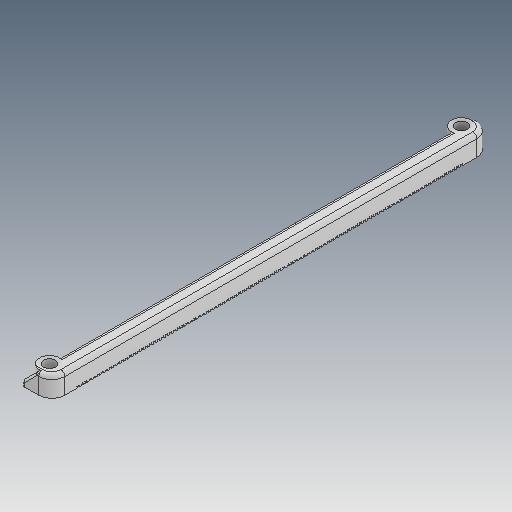
# Autodesk Inventor part: front_panel_mount_end
Saved by Autodesk Inventor 2027 (Build 310192060, 192F)
## iProperties
Created: 2026-07-28
Part Number: front_panel_mount_end
Material: Generic
Document SubType Name: Modeling
Designer: prest
Density: 1 g/cm^3
Appearance: Default
Author: prest
Autodesk Inventor part; units mm, degrees
ref_plane "YZ Plane" through (0, 0, 0) normal (1, 0, 0) x (0, 1, 0)
ref_plane "XZ Plane" through (0, 0, 0) normal (0, 1, 0) x (-1, 0, 0)
ref_plane "XY Plane" through (0, 0, 0) normal (0, 0, 1) x (1, 0, 0)
sketch "Sketch1" plane through (0, 0, 0) normal (0, 1, 0) x (-1, 0, 0)
  line L0 (7.375, 108.5) -> (-7.375, 108.5)
  line L1 (-7.375, 108.5) -> (-7.375, -108.5)
  line L2 (-7.375, -108.5) -> (7.375, -108.5)
  line L3 (7.375, -108.5) -> (7.375, 108.5)
  point P0 (0, 0)
  point P1 (0, 108.5)
  point P2 (7.375, 0)
  dimension "d0" = 217
  dimension "d1" = 14.75
  constraints: 8 end point, 2 midpoint, 2 parallel, 1 horizontal, 1 horizontal alignment, 1 perpendicular, 1 vertical alignment
  measures "d0" distance of L2.end L0.start
  measures "d1" distance of L0.start L0.end
extrude "Extrusion1" add sketch "Sketch1" along normal blind 10
chamfer "Chamfer1" distance 8 angle 45 1 edges at (-7.375, 10, 0)
sketch "Sketch2" plane through (0, 0, 0) normal (0, -1, 0) x (1, 0, 0)
  line L0 (-7.375, -108.5) -> (-7.375, 108.5) projected
  point P0 (0, 0)
  point P1 (0.068, -101.6793)
  point P2 (0.068, 102.3207)
  point P3 (-7.375, -108.4123)
  point P4 (-7.375, 108.4123)
  dimension "d10" = 204
  dimension "d11" = 7.443
  constraints: 1 vertical alignment
  measures "d10" distance of point (0.068, -101.679) point (0.068, 102.321)
  measures "d11" distance from line of L0 point (0.068, 102.321)
hole "Hole1" at (0.068, 0, -101.6793) at (0.068, 0, 102.3207) direction (0, 1, 0) diameter 6 end through all
sketch "Sketch3" plane through (0, 0, 0) normal (0, -1, 0) x (1, 0, 0)
  arc A0 (0.625, -98.7315) -> (0.625, -104.6271) centre (0.068, -101.6793) ccw projected
  circle A1 centre (0.068, -101.6793) radius 3
  circle A2 centre (0.068, -101.6793) radius 5
  circle A3 centre (0.068, 102.3207) radius 3 projected
  circle A4 centre (0.068, 102.3207) radius 5
  point P0 (0, 0)
  point P1 (0.0392, -98.6794)
  point P2 (0.0392, -104.6792)
  point P3 (0.0392, -104.6792)
  point P4 (0.0392, -98.6794)
  dimension "d19" = 10
  dimension "d20" = 10
  constraints: 3 centre point, 3 coincident
  measures "d19" diameter of A2
  measures "d20" diameter of A4
extrude "Extrusion2" add sketch "Sketch3" against normal blind 10
fillet "Fillet5" radius 6.5 2 edges at (7.375, 5, 108.5) (7.375, 5, -108.5)
fillet "Fillet6" radius 2 6 edges at (0.75, 10, 108.5) (7.375, 10, 0) (5.4712, 10, -106.5962) (0.75, 10, -108.5) (5.4712, 10, 106.5962) (0.625, 10, 0.3207)
fillet "Fillet7" radius 2 1 edges at (-7.375, 2, 0)
fillet "Fillet8" radius 1 8 edges at (-0.2821, 9.0929, 108.175) (-7.2228, 1.9369, 108.5) (-7.375, 0.5858, 108.5) (-4.0821, 5.2929, 108.5) (-7.2228, 1.9369, -108.5) (-7.375, 0.5858, -108.5) (-0.0144, 9.3606, -107.9659) (-4.0821, 5.2929, -108.5)
sketch "Sketch4" plane through (0.0392, 9.4142, -96.6794) normal (-0.7071068, 0.7071068, 0) x (-0.7071068, -0.7071068, 0)
  line L0 (8.6569, 192.6794) -> (1, 192.6794)
  line L1 (1, 191.6794) -> (8.6569, 191.6794)
  line L2 (8.6569, 191.6794) -> (8.6569, 192.6794)
  line L3 (1, 192.6794) -> (1, 191.6794)
  line L4 (1, -11.8206) -> (9.6569, -11.8206) projected
  ellipse E0 centre (6.6365, -4.9999) end of major axis (6.6365, -7.9999) minor radius 2.1213 projected
  line L5 (-6.7225, 1.1794) -> (12.4454, 1.1794) construction
  line L6 (11.8995, -10.8206) -> (11.8995, 204.1794) projected
  line L7 (9.6569, 205.1794) -> (1, 205.1794) projected
  line L8 (0, 0) -> (0, 194.0002) projected
  line L9 (9.6569, 204.1794) -> (9.6569, -10.8206) projected
  line L10 (8.6569, 190.6794) -> (1, 190.6794)
  line L11 (8.6569, 189.6794) -> (8.6569, 190.6794)
  line L12 (1, 189.6794) -> (8.6569, 189.6794)
  line L13 (1, 190.6794) -> (1, 189.6794)
  line L14 (8.6569, 188.6794) -> (1, 188.6794)
  line L15 (8.6569, 187.6794) -> (8.6569, 188.6794)
  line L16 (1, 187.6794) -> (8.6569, 187.6794)
  line L17 (1, 188.6794) -> (1, 187.6794)
  line L18 (8.6569, 186.6794) -> (1, 186.6794)
  line L19 (8.6569, 185.6794) -> (8.6569, 186.6794)
  line L20 (1, 185.6794) -> (8.6569, 185.6794)
  line L21 (1, 186.6794) -> (1, 185.6794)
  line L22 (8.6569, 184.6794) -> (1, 184.6794)
  line L23 (8.6569, 183.6794) -> (8.6569, 184.6794)
  line L24 (1, 183.6794) -> (8.6569, 183.6794)
  line L25 (1, 184.6794) -> (1, 183.6794)
  line L26 (8.6569, 182.6794) -> (1, 182.6794)
  line L27 (8.6569, 181.6794) -> (8.6569, 182.6794)
  line L28 (1, 181.6794) -> (8.6569, 181.6794)
  line L29 (1, 182.6794) -> (1, 181.6794)
  line L30 (8.6569, 180.6794) -> (1, 180.6794)
  line L31 (8.6569, 179.6794) -> (8.6569, 180.6794)
  line L32 (1, 179.6794) -> (8.6569, 179.6794)
  line L33 (1, 180.6794) -> (1, 179.6794)
  line L34 (8.6569, 178.6794) -> (1, 178.6794)
  line L35 (8.6569, 177.6794) -> (8.6569, 178.6794)
  line L36 (1, 177.6794) -> (8.6569, 177.6794)
  line L37 (1, 178.6794) -> (1, 177.6794)
  line L38 (8.6569, 176.6794) -> (1, 176.6794)
  line L39 (8.6569, 175.6794) -> (8.6569, 176.6794)
  line L40 (1, 175.6794) -> (8.6569, 175.6794)
  line L41 (1, 176.6794) -> (1, 175.6794)
  line L42 (8.6569, 174.6794) -> (1, 174.6794)
  line L43 (8.6569, 173.6794) -> (8.6569, 174.6794)
  line L44 (1, 173.6794) -> (8.6569, 173.6794)
  line L45 (1, 174.6794) -> (1, 173.6794)
  line L46 (8.6569, 172.6794) -> (1, 172.6794)
  line L47 (8.6569, 171.6794) -> (8.6569, 172.6794)
  line L48 (1, 171.6794) -> (8.6569, 171.6794)
  line L49 (1, 172.6794) -> (1, 171.6794)
  line L50 (8.6569, 170.6794) -> (1, 170.6794)
  line L51 (8.6569, 169.6794) -> (8.6569, 170.6794)
  line L52 (1, 169.6794) -> (8.6569, 169.6794)
  line L53 (1, 170.6794) -> (1, 169.6794)
  line L54 (8.6569, 168.6794) -> (1, 168.6794)
  line L55 (8.6569, 167.6794) -> (8.6569, 168.6794)
  line L56 (1, 167.6794) -> (8.6569, 167.6794)
  line L57 (1, 168.6794) -> (1, 167.6794)
  line L58 (8.6569, 166.6794) -> (1, 166.6794)
  line L59 (8.6569, 165.6794) -> (8.6569, 166.6794)
  line L60 (1, 165.6794) -> (8.6569, 165.6794)
  line L61 (1, 166.6794) -> (1, 165.6794)
  line L62 (8.6569, 164.6794) -> (1, 164.6794)
  line L63 (8.6569, 163.6794) -> (8.6569, 164.6794)
  line L64 (1, 163.6794) -> (8.6569, 163.6794)
  line L65 (1, 164.6794) -> (1, 163.6794)
  line L66 (8.6569, 162.6794) -> (1, 162.6794)
  line L67 (8.6569, 161.6794) -> (8.6569, 162.6794)
  line L68 (1, 161.6794) -> (8.6569, 161.6794)
  line L69 (1, 162.6794) -> (1, 161.6794)
  line L70 (8.6569, 160.6794) -> (1, 160.6794)
  line L71 (8.6569, 159.6794) -> (8.6569, 160.6794)
  line L72 (1, 159.6794) -> (8.6569, 159.6794)
  line L73 (1, 160.6794) -> (1, 159.6794)
  line L74 (8.6569, 158.6794) -> (1, 158.6794)
  line L75 (8.6569, 157.6794) -> (8.6569, 158.6794)
  line L76 (1, 157.6794) -> (8.6569, 157.6794)
  line L77 (1, 158.6794) -> (1, 157.6794)
  line L78 (8.6569, 156.6794) -> (1, 156.6794)
  line L79 (8.6569, 155.6794) -> (8.6569, 156.6794)
  line L80 (1, 155.6794) -> (8.6569, 155.6794)
  line L81 (1, 156.6794) -> (1, 155.6794)
  line L82 (8.6569, 154.6794) -> (1, 154.6794)
  line L83 (8.6569, 153.6794) -> (8.6569, 154.6794)
  line L84 (1, 153.6794) -> (8.6569, 153.6794)
  line L85 (1, 154.6794) -> (1, 153.6794)
  line L86 (8.6569, 152.6794) -> (1, 152.6794)
  line L87 (8.6569, 151.6794) -> (8.6569, 152.6794)
  line L88 (1, 151.6794) -> (8.6569, 151.6794)
  line L89 (1, 152.6794) -> (1, 151.6794)
  line L90 (8.6569, 150.6794) -> (1, 150.6794)
  line L91 (8.6569, 149.6794) -> (8.6569, 150.6794)
  line L92 (1, 149.6794) -> (8.6569, 149.6794)
  line L93 (1, 150.6794) -> (1, 149.6794)
  line L94 (8.6569, 148.6794) -> (1, 148.6794)
  line L95 (8.6569, 147.6794) -> (8.6569, 148.6794)
  line L96 (1, 147.6794) -> (8.6569, 147.6794)
  line L97 (1, 148.6794) -> (1, 147.6794)
  line L98 (8.6569, 146.6794) -> (1, 146.6794)
  line L99 (8.6569, 145.6794) -> (8.6569, 146.6794)
  line L100 (1, 145.6794) -> (8.6569, 145.6794)
  line L101 (1, 146.6794) -> (1, 145.6794)
  line L102 (8.6569, 144.6794) -> (1, 144.6794)
  line L103 (8.6569, 143.6794) -> (8.6569, 144.6794)
  line L104 (1, 143.6794) -> (8.6569, 143.6794)
  line L105 (1, 144.6794) -> (1, 143.6794)
  line L106 (8.6569, 142.6794) -> (1, 142.6794)
  line L107 (8.6569, 141.6794) -> (8.6569, 142.6794)
  line L108 (1, 141.6794) -> (8.6569, 141.6794)
  line L109 (1, 142.6794) -> (1, 141.6794)
  line L110 (8.6569, 140.6794) -> (1, 140.6794)
  line L111 (8.6569, 139.6794) -> (8.6569, 140.6794)
  line L112 (1, 139.6794) -> (8.6569, 139.6794)
  line L113 (1, 140.6794) -> (1, 139.6794)
  line L114 (8.6569, 138.6794) -> (1, 138.6794)
  line L115 (8.6569, 137.6794) -> (8.6569, 138.6794)
  line L116 (1, 137.6794) -> (8.6569, 137.6794)
  line L117 (1, 138.6794) -> (1, 137.6794)
  line L118 (8.6569, 136.6794) -> (1, 136.6794)
  line L119 (8.6569, 135.6794) -> (8.6569, 136.6794)
  line L120 (1, 135.6794) -> (8.6569, 135.6794)
  line L121 (1, 136.6794) -> (1, 135.6794)
  line L122 (8.6569, 134.6794) -> (1, 134.6794)
  line L123 (8.6569, 133.6794) -> (8.6569, 134.6794)
  line L124 (1, 133.6794) -> (8.6569, 133.6794)
  line L125 (1, 134.6794) -> (1, 133.6794)
  line L126 (8.6569, 132.6794) -> (1, 132.6794)
  line L127 (8.6569, 131.6794) -> (8.6569, 132.6794)
  line L128 (1, 131.6794) -> (8.6569, 131.6794)
  line L129 (1, 132.6794) -> (1, 131.6794)
  line L130 (8.6569, 130.6794) -> (1, 130.6794)
  line L131 (8.6569, 129.6794) -> (8.6569, 130.6794)
  line L132 (1, 129.6794) -> (8.6569, 129.6794)
  line L133 (1, 130.6794) -> (1, 129.6794)
  line L134 (8.6569, 128.6794) -> (1, 128.6794)
  line L135 (8.6569, 127.6794) -> (8.6569, 128.6794)
  line L136 (1, 127.6794) -> (8.6569, 127.6794)
  line L137 (1, 128.6794) -> (1, 127.6794)
  line L138 (8.6569, 126.6794) -> (1, 126.6794)
  line L139 (8.6569, 125.6794) -> (8.6569, 126.6794)
  line L140 (1, 125.6794) -> (8.6569, 125.6794)
  line L141 (1, 126.6794) -> (1, 125.6794)
  line L142 (8.6569, 124.6794) -> (1, 124.6794)
  line L143 (8.6569, 123.6794) -> (8.6569, 124.6794)
  line L144 (1, 123.6794) -> (8.6569, 123.6794)
  line L145 (1, 124.6794) -> (1, 123.6794)
  line L146 (8.6569, 122.6794) -> (1, 122.6794)
  line L147 (8.6569, 121.6794) -> (8.6569, 122.6794)
  line L148 (1, 121.6794) -> (8.6569, 121.6794)
  line L149 (1, 122.6794) -> (1, 121.6794)
  line L150 (8.6569, 120.6794) -> (1, 120.6794)
  line L151 (8.6569, 119.6794) -> (8.6569, 120.6794)
  line L152 (1, 119.6794) -> (8.6569, 119.6794)
  line L153 (1, 120.6794) -> (1, 119.6794)
  line L154 (8.6569, 118.6794) -> (1, 118.6794)
  line L155 (8.6569, 117.6794) -> (8.6569, 118.6794)
  line L156 (1, 117.6794) -> (8.6569, 117.6794)
  line L157 (1, 118.6794) -> (1, 117.6794)
  line L158 (8.6569, 116.6794) -> (1, 116.6794)
  line L159 (8.6569, 115.6794) -> (8.6569, 116.6794)
  line L160 (1, 115.6794) -> (8.6569, 115.6794)
  line L161 (1, 116.6794) -> (1, 115.6794)
  line L162 (8.6569, 114.6794) -> (1, 114.6794)
  line L163 (8.6569, 113.6794) -> (8.6569, 114.6794)
  line L164 (1, 113.6794) -> (8.6569, 113.6794)
  line L165 (1, 114.6794) -> (1, 113.6794)
  line L166 (8.6569, 112.6794) -> (1, 112.6794)
  line L167 (8.6569, 111.6794) -> (8.6569, 112.6794)
  line L168 (1, 111.6794) -> (8.6569, 111.6794)
  line L169 (1, 112.6794) -> (1, 111.6794)
  line L170 (8.6569, 110.6794) -> (1, 110.6794)
  line L171 (8.6569, 109.6794) -> (8.6569, 110.6794)
  line L172 (1, 109.6794) -> (8.6569, 109.6794)
  line L173 (1, 110.6794) -> (1, 109.6794)
  line L174 (8.6569, 108.6794) -> (1, 108.6794)
  line L175 (8.6569, 107.6794) -> (8.6569, 108.6794)
  line L176 (1, 107.6794) -> (8.6569, 107.6794)
  line L177 (1, 108.6794) -> (1, 107.6794)
  line L178 (8.6569, 106.6794) -> (1, 106.6794)
  line L179 (8.6569, 105.6794) -> (8.6569, 106.6794)
  line L180 (1, 105.6794) -> (8.6569, 105.6794)
  line L181 (1, 106.6794) -> (1, 105.6794)
  line L182 (8.6569, 104.6794) -> (1, 104.6794)
  line L183 (8.6569, 103.6794) -> (8.6569, 104.6794)
  line L184 (1, 103.6794) -> (8.6569, 103.6794)
  line L185 (1, 104.6794) -> (1, 103.6794)
  line L186 (8.6569, 102.6794) -> (1, 102.6794)
  line L187 (8.6569, 101.6794) -> (8.6569, 102.6794)
  line L188 (1, 101.6794) -> (8.6569, 101.6794)
  line L189 (1, 102.6794) -> (1, 101.6794)
  line L190 (8.6569, 100.6794) -> (1, 100.6794)
  line L191 (8.6569, 99.6794) -> (8.6569, 100.6794)
  line L192 (1, 99.6794) -> (8.6569, 99.6794)
  line L193 (1, 100.6794) -> (1, 99.6794)
  line L194 (8.6569, 98.6794) -> (1, 98.6794)
  line L195 (8.6569, 97.6794) -> (8.6569, 98.6794)
  line L196 (1, 97.6794) -> (8.6569, 97.6794)
  line L197 (1, 98.6794) -> (1, 97.6794)
  line L198 (8.6569, 96.6794) -> (1, 96.6794)
  line L199 (8.6569, 95.6794) -> (8.6569, 96.6794)
  line L200 (1, 95.6794) -> (8.6569, 95.6794)
  line L201 (1, 96.6794) -> (1, 95.6794)
  line L202 (8.6569, 94.6794) -> (1, 94.6794)
  line L203 (8.6569, 93.6794) -> (8.6569, 94.6794)
  line L204 (1, 93.6794) -> (8.6569, 93.6794)
  line L205 (1, 94.6794) -> (1, 93.6794)
  line L206 (8.6569, 92.6794) -> (1, 92.6794)
  line L207 (8.6569, 91.6794) -> (8.6569, 92.6794)
  line L208 (1, 91.6794) -> (8.6569, 91.6794)
  line L209 (1, 92.6794) -> (1, 91.6794)
  line L210 (8.6569, 90.6794) -> (1, 90.6794)
  line L211 (8.6569, 89.6794) -> (8.6569, 90.6794)
  line L212 (1, 89.6794) -> (8.6569, 89.6794)
  line L213 (1, 90.6794) -> (1, 89.6794)
  line L214 (8.6569, 88.6794) -> (1, 88.6794)
  line L215 (8.6569, 87.6794) -> (8.6569, 88.6794)
  line L216 (1, 87.6794) -> (8.6569, 87.6794)
  line L217 (1, 88.6794) -> (1, 87.6794)
  line L218 (8.6569, 86.6794) -> (1, 86.6794)
  line L219 (8.6569, 85.6794) -> (8.6569, 86.6794)
  line L220 (1, 85.6794) -> (8.6569, 85.6794)
  line L221 (1, 86.6794) -> (1, 85.6794)
  line L222 (8.6569, 84.6794) -> (1, 84.6794)
  line L223 (8.6569, 83.6794) -> (8.6569, 84.6794)
  line L224 (1, 83.6794) -> (8.6569, 83.6794)
  line L225 (1, 84.6794) -> (1, 83.6794)
  line L226 (8.6569, 82.6794) -> (1, 82.6794)
  line L227 (8.6569, 81.6794) -> (8.6569, 82.6794)
  line L228 (1, 81.6794) -> (8.6569, 81.6794)
  line L229 (1, 82.6794) -> (1, 81.6794)
  line L230 (8.6569, 80.6794) -> (1, 80.6794)
  line L231 (8.6569, 79.6794) -> (8.6569, 80.6794)
  line L232 (1, 79.6794) -> (8.6569, 79.6794)
  line L233 (1, 80.6794) -> (1, 79.6794)
  line L234 (8.6569, 78.6794) -> (1, 78.6794)
  line L235 (8.6569, 77.6794) -> (8.6569, 78.6794)
  line L236 (1, 77.6794) -> (8.6569, 77.6794)
  line L237 (1, 78.6794) -> (1, 77.6794)
  line L238 (8.6569, 76.6794) -> (1, 76.6794)
  line L239 (8.6569, 75.6794) -> (8.6569, 76.6794)
  line L240 (1, 75.6794) -> (8.6569, 75.6794)
  line L241 (1, 76.6794) -> (1, 75.6794)
  line L242 (8.6569, 74.6794) -> (1, 74.6794)
  line L243 (8.6569, 73.6794) -> (8.6569, 74.6794)
  line L244 (1, 73.6794) -> (8.6569, 73.6794)
  line L245 (1, 74.6794) -> (1, 73.6794)
  line L246 (8.6569, 72.6794) -> (1, 72.6794)
  line L247 (8.6569, 71.6794) -> (8.6569, 72.6794)
  line L248 (1, 71.6794) -> (8.6569, 71.6794)
  line L249 (1, 72.6794) -> (1, 71.6794)
  line L250 (8.6569, 70.6794) -> (1, 70.6794)
  line L251 (8.6569, 69.6794) -> (8.6569, 70.6794)
  line L252 (1, 69.6794) -> (8.6569, 69.6794)
  line L253 (1, 70.6794) -> (1, 69.6794)
  line L254 (8.6569, 68.6794) -> (1, 68.6794)
  line L255 (8.6569, 67.6794) -> (8.6569, 68.6794)
  line L256 (1, 67.6794) -> (8.6569, 67.6794)
  line L257 (1, 68.6794) -> (1, 67.6794)
  line L258 (8.6569, 66.6794) -> (1, 66.6794)
  line L259 (8.6569, 65.6794) -> (8.6569, 66.6794)
  line L260 (1, 65.6794) -> (8.6569, 65.6794)
  line L261 (1, 66.6794) -> (1, 65.6794)
  line L262 (8.6569, 64.6794) -> (1, 64.6794)
  line L263 (8.6569, 63.6794) -> (8.6569, 64.6794)
  line L264 (1, 63.6794) -> (8.6569, 63.6794)
  line L265 (1, 64.6794) -> (1, 63.6794)
  line L266 (8.6569, 62.6794) -> (1, 62.6794)
  line L267 (8.6569, 61.6794) -> (8.6569, 62.6794)
  line L268 (1, 61.6794) -> (8.6569, 61.6794)
  line L269 (1, 62.6794) -> (1, 61.6794)
  line L270 (8.6569, 60.6794) -> (1, 60.6794)
  line L271 (8.6569, 59.6794) -> (8.6569, 60.6794)
  line L272 (1, 59.6794) -> (8.6569, 59.6794)
  line L273 (1, 60.6794) -> (1, 59.6794)
  line L274 (8.6569, 58.6794) -> (1, 58.6794)
  line L275 (8.6569, 57.6794) -> (8.6569, 58.6794)
  line L276 (1, 57.6794) -> (8.6569, 57.6794)
  line L277 (1, 58.6794) -> (1, 57.6794)
  line L278 (8.6569, 56.6794) -> (1, 56.6794)
  line L279 (8.6569, 55.6794) -> (8.6569, 56.6794)
  line L280 (1, 55.6794) -> (8.6569, 55.6794)
  line L281 (1, 56.6794) -> (1, 55.6794)
  line L282 (8.6569, 54.6794) -> (1, 54.6794)
  line L283 (8.6569, 53.6794) -> (8.6569, 54.6794)
  line L284 (1, 53.6794) -> (8.6569, 53.6794)
  line L285 (1, 54.6794) -> (1, 53.6794)
  line L286 (8.6569, 52.6794) -> (1, 52.6794)
  line L287 (8.6569, 51.6794) -> (8.6569, 52.6794)
  line L288 (1, 51.6794) -> (8.6569, 51.6794)
  line L289 (1, 52.6794) -> (1, 51.6794)
  line L290 (8.6569, 50.6794) -> (1, 50.6794)
  line L291 (8.6569, 49.6794) -> (8.6569, 50.6794)
  line L292 (1, 49.6794) -> (8.6569, 49.6794)
  line L293 (1, 50.6794) -> (1, 49.6794)
  line L294 (8.6569, 48.6794) -> (1, 48.6794)
  line L295 (8.6569, 47.6794) -> (8.6569, 48.6794)
  line L296 (1, 47.6794) -> (8.6569, 47.6794)
  line L297 (1, 48.6794) -> (1, 47.6794)
  line L298 (8.6569, 46.6794) -> (1, 46.6794)
  line L299 (8.6569, 45.6794) -> (8.6569, 46.6794)
  line L300 (1, 45.6794) -> (8.6569, 45.6794)
  line L301 (1, 46.6794) -> (1, 45.6794)
  line L302 (8.6569, 44.6794) -> (1, 44.6794)
  line L303 (8.6569, 43.6794) -> (8.6569, 44.6794)
  line L304 (1, 43.6794) -> (8.6569, 43.6794)
  line L305 (1, 44.6794) -> (1, 43.6794)
  line L306 (8.6569, 42.6794) -> (1, 42.6794)
  line L307 (8.6569, 41.6794) -> (8.6569, 42.6794)
  line L308 (1, 41.6794) -> (8.6569, 41.6794)
  line L309 (1, 42.6794) -> (1, 41.6794)
  line L310 (8.6569, 40.6794) -> (1, 40.6794)
  line L311 (8.6569, 39.6794) -> (8.6569, 40.6794)
  line L312 (1, 39.6794) -> (8.6569, 39.6794)
  line L313 (1, 40.6794) -> (1, 39.6794)
  line L314 (8.6569, 38.6794) -> (1, 38.6794)
  line L315 (8.6569, 37.6794) -> (8.6569, 38.6794)
  line L316 (1, 37.6794) -> (8.6569, 37.6794)
  line L317 (1, 38.6794) -> (1, 37.6794)
  line L318 (8.6569, 36.6794) -> (1, 36.6794)
  line L319 (8.6569, 35.6794) -> (8.6569, 36.6794)
  line L320 (1, 35.6794) -> (8.6569, 35.6794)
  line L321 (1, 36.6794) -> (1, 35.6794)
  line L322 (8.6569, 34.6794) -> (1, 34.6794)
  line L323 (8.6569, 33.6794) -> (8.6569, 34.6794)
  line L324 (1, 33.6794) -> (8.6569, 33.6794)
  line L325 (1, 34.6794) -> (1, 33.6794)
  line L326 (8.6569, 32.6794) -> (1, 32.6794)
  line L327 (8.6569, 31.6794) -> (8.6569, 32.6794)
  line L328 (1, 31.6794) -> (8.6569, 31.6794)
  line L329 (1, 32.6794) -> (1, 31.6794)
  line L330 (8.6569, 30.6794) -> (1, 30.6794)
  line L331 (8.6569, 29.6794) -> (8.6569, 30.6794)
  line L332 (1, 29.6794) -> (8.6569, 29.6794)
  line L333 (1, 30.6794) -> (1, 29.6794)
  line L334 (8.6569, 28.6794) -> (1, 28.6794)
  line L335 (8.6569, 27.6794) -> (8.6569, 28.6794)
  line L336 (1, 27.6794) -> (8.6569, 27.6794)
  line L337 (1, 28.6794) -> (1, 27.6794)
  line L338 (8.6569, 26.6794) -> (1, 26.6794)
  line L339 (8.6569, 25.6794) -> (8.6569, 26.6794)
  line L340 (1, 25.6794) -> (8.6569, 25.6794)
  line L341 (1, 26.6794) -> (1, 25.6794)
  line L342 (8.6569, 24.6794) -> (1, 24.6794)
  line L343 (8.6569, 23.6794) -> (8.6569, 24.6794)
  line L344 (1, 23.6794) -> (8.6569, 23.6794)
  line L345 (1, 24.6794) -> (1, 23.6794)
  line L346 (8.6569, 22.6794) -> (1, 22.6794)
  line L347 (8.6569, 21.6794) -> (8.6569, 22.6794)
  line L348 (1, 21.6794) -> (8.6569, 21.6794)
  line L349 (1, 22.6794) -> (1, 21.6794)
  line L350 (8.6569, 20.6794) -> (1, 20.6794)
  line L351 (8.6569, 19.6794) -> (8.6569, 20.6794)
  line L352 (1, 19.6794) -> (8.6569, 19.6794)
  line L353 (1, 20.6794) -> (1, 19.6794)
  line L354 (8.6569, 18.6794) -> (1, 18.6794)
  line L355 (8.6569, 17.6794) -> (8.6569, 18.6794)
  line L356 (1, 17.6794) -> (8.6569, 17.6794)
  line L357 (1, 18.6794) -> (1, 17.6794)
  line L358 (8.6569, 16.6794) -> (1, 16.6794)
  line L359 (8.6569, 15.6794) -> (8.6569, 16.6794)
  line L360 (1, 15.6794) -> (8.6569, 15.6794)
  line L361 (1, 16.6794) -> (1, 15.6794)
  line L362 (8.6569, 14.6794) -> (1, 14.6794)
  line L363 (8.6569, 13.6794) -> (8.6569, 14.6794)
  line L364 (1, 13.6794) -> (8.6569, 13.6794)
  line L365 (1, 14.6794) -> (1, 13.6794)
  line L366 (8.6569, 12.6794) -> (1, 12.6794)
  line L367 (8.6569, 11.6794) -> (8.6569, 12.6794)
  line L368 (1, 11.6794) -> (8.6569, 11.6794)
  line L369 (1, 12.6794) -> (1, 11.6794)
  line L370 (8.6569, 10.6794) -> (1, 10.6794)
  line L371 (8.6569, 9.6794) -> (8.6569, 10.6794)
  line L372 (1, 9.6794) -> (8.6569, 9.6794)
  line L373 (1, 10.6794) -> (1, 9.6794)
  line L374 (8.6569, 8.6794) -> (1, 8.6794)
  line L375 (8.6569, 7.6794) -> (8.6569, 8.6794)
  line L376 (1, 7.6794) -> (8.6569, 7.6794)
  line L377 (1, 8.6794) -> (1, 7.6794)
  line L378 (8.6569, 6.6794) -> (1, 6.6794)
  line L379 (8.6569, 5.6794) -> (8.6569, 6.6794)
  line L380 (1, 5.6794) -> (8.6569, 5.6794)
  line L381 (1, 6.6794) -> (1, 5.6794)
  line L382 (8.6569, 4.6794) -> (1, 4.6794)
  line L383 (8.6569, 3.6794) -> (8.6569, 4.6794)
  line L384 (1, 3.6794) -> (8.6569, 3.6794)
  line L385 (1, 4.6794) -> (1, 3.6794)
  line L386 (8.6569, 2.6794) -> (1, 2.6794)
  line L387 (8.6569, 1.6794) -> (8.6569, 2.6794)
  line L388 (1, 1.6794) -> (8.6569, 1.6794)
  line L389 (1, 2.6794) -> (1, 1.6794)
  point P0 (6.6846, 96.6794)
  point P1 (8.6569, 192.1794)
  point P2 (8.6569, 190.1794)
  point P3 (8.6569, 188.1794)
  point P4 (8.6569, 186.1794)
  point P5 (8.6569, 184.1794)
  point P6 (8.6569, 182.1794)
  point P7 (8.6569, 180.1794)
  point P8 (8.6569, 178.1794)
  point P9 (8.6569, 176.1794)
  point P10 (8.6569, 174.1794)
  point P11 (8.6569, 172.1794)
  point P12 (8.6569, 170.1794)
  point P13 (8.6569, 168.1794)
  point P14 (8.6569, 166.1794)
  point P15 (8.6569, 164.1794)
  point P16 (8.6569, 162.1794)
  point P17 (8.6569, 160.1794)
  point P18 (8.6569, 158.1794)
  point P19 (8.6569, 156.1794)
  point P20 (8.6569, 154.1794)
  point P21 (8.6569, 152.1794)
  point P22 (8.6569, 150.1794)
  point P23 (8.6569, 148.1794)
  point P24 (8.6569, 146.1794)
  point P25 (8.6569, 144.1794)
  point P26 (8.6569, 142.1794)
  point P27 (8.6569, 140.1794)
  point P28 (8.6569, 138.1794)
  point P29 (8.6569, 136.1794)
  point P30 (8.6569, 134.1794)
  point P31 (8.6569, 132.1794)
  point P32 (8.6569, 130.1794)
  point P33 (8.6569, 128.1794)
  point P34 (8.6569, 126.1794)
  point P35 (8.6569, 124.1794)
  point P36 (8.6569, 122.1794)
  point P37 (8.6569, 120.1794)
  point P38 (8.6569, 118.1794)
  point P39 (8.6569, 116.1794)
  point P40 (8.6569, 114.1794)
  point P41 (8.6569, 112.1794)
  point P42 (8.6569, 110.1794)
  point P43 (8.6569, 108.1794)
  point P44 (8.6569, 106.1794)
  point P45 (8.6569, 104.1794)
  point P46 (8.6569, 102.1794)
  point P47 (8.6569, 100.1794)
  point P48 (8.6569, 98.1794)
  point P49 (8.6569, 96.1794)
  point P50 (8.6569, 94.1794)
  point P51 (8.6569, 92.1794)
  point P52 (8.6569, 90.1794)
  point P53 (8.6569, 88.1794)
  point P54 (8.6569, 86.1794)
  point P55 (8.6569, 84.1794)
  point P56 (8.6569, 82.1794)
  point P57 (8.6569, 80.1794)
  point P58 (8.6569, 78.1794)
  point P59 (8.6569, 76.1794)
  point P60 (8.6569, 74.1794)
  point P61 (8.6569, 72.1794)
  point P62 (8.6569, 70.1794)
  point P63 (8.6569, 68.1794)
  point P64 (8.6569, 66.1794)
  point P65 (8.6569, 64.1794)
  point P66 (8.6569, 62.1794)
  point P67 (8.6569, 60.1794)
  point P68 (8.6569, 58.1794)
  point P69 (8.6569, 56.1794)
  point P70 (8.6569, 54.1794)
  point P71 (8.6569, 52.1794)
  point P72 (8.6569, 50.1794)
  point P73 (8.6569, 48.1794)
  point P74 (8.6569, 46.1794)
  point P75 (8.6569, 44.1794)
  point P76 (8.6569, 42.1794)
  point P77 (8.6569, 40.1794)
  point P78 (8.6569, 38.1794)
  point P79 (8.6569, 36.1794)
  point P80 (8.6569, 34.1794)
  point P81 (8.6569, 32.1794)
  point P82 (8.6569, 30.1794)
  point P83 (8.6569, 28.1794)
  point P84 (8.6569, 26.1794)
  point P85 (8.6569, 24.1794)
  point P86 (8.6569, 22.1794)
  point P87 (8.6569, 20.1794)
  point P88 (8.6569, 18.1794)
  point P89 (8.6569, 16.1794)
  point P90 (8.6569, 14.1794)
  point P91 (8.6569, 12.1794)
  point P92 (8.6569, 10.1794)
  point P93 (8.6569, 8.1794)
  point P94 (8.6569, 6.1794)
  point P95 (8.6569, 4.1794)
  point P96 (8.6569, 2.1794)
  dimension "d28" = 1
  dimension "d31" = 13
  dimension "d32" = 13
  dimension "d34" = 1
  dimension "d35" = 1
  dimension "d38" = 2
  constraints: 770 end point, 2 horizontal, 2 perpendicular, 1 midpoint, 1 vertical, 855 other
  measures "d28" distance of L1.end L0.start
  measures "d31" distance between parallel lines of L4 L5
  measures "d32" distance from line of point (8.657, 192.179) L7
  measures "d34" distance between parallel lines of L8 L3
  measures "d35" distance between parallel lines of L9 L2
  measures "d38" distance of L0.start L10.start
extrude "Extrusion3" cut sketch "Sketch4" against normal through all contours L2 L1 L3 L0 | L11 L12 L13 L10 | L15 L16 L17 L14 | L19 L20 L21 L18 | L23 L24 L25 L22 | L27 L28 L29 L26 | L31 L32 L33 L30 | L35 L36 L37 L34 | L39 L40 L41 L38 | L43 L44 L45 L42 | L47 L48 L49 L46 | L51 L52 L53 L50 | L55 L56 L57 L54 | L59 L60 L61 L58 | L63 L64 L65 L62 | L67 L68 L69 L66 | L71 L72 L73 L70 | L75 L76 L77 L74 | L79 L80 L81 L78 | L83 L84 L85 L82 | L87 L88 L89 L86 | L91 L92 L93 L90 | L95 L96 L97 L94 | L99 L100 L101 L98 | L103 L104 L105 L102 | L107 L108 L109 L106 | L111 L112 L113 L110 | L115 L116 L117 L114 | L119 L120 L121 L118 | L123 L124 L125 L122 | L127 L128 L129 L126 | L131 L132 L133 L130 | L135 L136 L137 L134 | L139 L140 L141 L138 | L143 L144 L145 L142 | L147 L148 L149 L146 | L151 L152 L153 L150 | L155 L156 L157 L154 | L159 L160 L161 L158 | L163 L164 L165 L162 | L167 L168 L169 L166 | L171 L172 L173 L170 | L175 L176 L177 L174 | L179 L180 L181 L178 | L183 L184 L185 L182 | L187 L188 L189 L186 | L191 L192 L193 L190 | L195 L196 L197 L194 | L199 L200 L201 L198 | L203 L204 L205 L202 | L207 L208 L209 L206 | L211 L212 L213 L210 | L215 L216 L217 L214 | L219 L220 L221 L218 | L223 L224 L225 L222 | L227 L228 L229 L226 | L231 L232 L233 L230 | L235 L236 L237 L234 | L239 L240 L241 L238 | L243 L244 L245 L242 | L247 L248 L249 L246 | L251 L252 L253 L250 | L255 L256 L257 L254 | L259 L260 L261 L258 | L263 L264 L265 L262 | L267 L268 L269 L266 | L271 L272 L273 L270 | L275 L276 L277 L274 | L279 L280 L281 L278 | L283 L284 L285 L282 | L287 L288 L289 L286 | L291 L292 L293 L290 | L295 L296 L297 L294 | L299 L300 L301 L298 | L303 L304 L305 L302 | L307 L308 L309 L306 | L311 L312 L313 L310 | L315 L316 L317 L314 | L319 L320 L321 L318 | L323 L324 L325 L322 | L327 L328 L329 L326 | L331 L332 L333 L330 | L335 L336 L337 L334 | L339 L340 L341 L338 | L343 L344 L345 L342 | L347 L348 L349 L346 | L351 L352 L353 L350 | L355 L356 L357 L354 | L359 L360 L361 L358 | L363 L364 L365 L362 | L367 L368 L369 L366 | L371 L372 L373 L370 | L375 L376 L377 L374 | L379 L380 L381 L378 | L383 L384 L385 L382 | L387 L388 L389 L386
equation "\"d35\" = d34"
body "Solid1"
